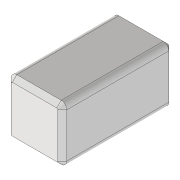
# Autodesk Inventor part: Motor
Saved by Autodesk Inventor 2020 (Build 240168000, 168)
## iProperties
Created: 2020-04-08
Part Number: Motor
Material: Generisch
Document SubType Name: Modeling
Designer: franz
Density: 1 g/cm^3
Appearance: Vorgabe
Author: franz
Autodesk Inventor part; units mm, degrees
ref_plane "YZ Plane" through (0, 0, 0) normal (1, 0, 0) x (0, 1, 0)
ref_plane "XZ Plane" through (0, 0, 0) normal (0, 1, 0) x (-1, 0, 0)
ref_plane "XY Plane" through (0, 0, 0) normal (0, 0, 1) x (1, 0, 0)
sketch "Skizze1" plane through (0, 0, 0) normal (0, 0, 1) x (1, 0, 0)
  line L0 (-40, -50) -> (40, -50)
  line L1 (50, -40) -> (50, 40)
  line L2 (40, 50) -> (-40, 50)
  line L3 (-50, 40) -> (-50, -40)
  line L4 (-50, -50) -> (50, 50) construction
  line L5 (50, -50) -> (-50, 50) construction
  arc A0 (-40, 50) -> (-50, 40) centre (-40, 40) ccw
  arc A1 (50, 40) -> (40, 50) centre (40, 40) ccw
  arc A2 (40, -50) -> (50, -40) centre (40, -40) ccw
  arc A3 (-50, -40) -> (-40, -50) centre (-40, -40) ccw
  point P0 (0, 0)
  dimension "d0" = 100
  dimension "d1" = 100
  dimension "d2" = 10
  constraints: 12 end point, 8 point on circle, 8 point on line, 8 tangent, 4 centre point, 3 equal radius, 2 midpoint, 2 parallel, 1 horizontal, 1 perpendicular
  measures "d0" distance of L5.end L4.end
  measures "d1" distance of L4.end L5.start
  measures "d2" radius of A0
extrude "Extrusion1" add sketch "Skizze1" along normal blind 200
chamfer "Fase1" distance 8 angle 45 16 edges at (50, 0, 200) (47.0711, 47.0711, 200) (0, 50, 200) (-47.0711, 47.0711, 200) (-50, 0, 200) (-47.0711, -47.0711, 200) (0, -50, 200) (47.0711, -47.0711, 200) (50, 0, 0) (47.0711, 47.0711, 0) (0, 50, 0) (-47.0711, 47.0711, 0) (-50, 0, 0) (-47.0711, -47.0711, 0) (0, -50, 0) (47.0711, -47.0711, 0)
